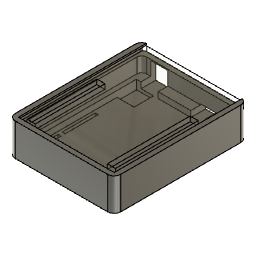
Projet fablabPORCEL (Autodesk Fusion 360 design; units mm, degrees)
Autodesk Fusion 360 part; units mm, degrees
sketch "Esquisse1" plane through (0, 0, 0) normal (0, 0, 1) x (1, 0, 0) in component "boite"
  line L0 (0, 0) -> (65, 0)
  line L1 (65, 0) -> (65, 82)
  line L2 (65, 82) -> (0, 82)
  line L3 (0, 82) -> (0, 0)
  dimension "d4" = 65
  dimension "d5" = 82
  constraint horizontal L0
  constraint vertical L1
  constraint horizontal L2
  constraint vertical L3
  constraint coincident L0.start L3.end
  measures "d4" distance of L0.start L0.end
  measures "d5" distance of L0.start L2.end
extrude "Extrusion1" add sketch "Esquisse1" along normal blind 20 makes body 1 in component "boite"
shell "Coque1" thickness 3 removed faces 1 at (21.6667, 54.6667, 20) on bodies 1 in component "boite"
sketch "Esquisse1 (2)" plane through (0, 0, 3) normal (0, 0, 1) x (-1, 0, 0) in component "boite"
  line L0 (-3, -79) -> (-3, -3)
  line L1 (-3, -3) -> (-62, -3)
  line L2 (-62, -3) -> (-62, -79)
  line L3 (-62, -79) -> (-3, -79)
  line L4 (-59.2367, -6.54) -> (-5.7633, -6.54) construction
  line L5 (-5.7633, -6.54) -> (-5.7633, -72.98)
  line L6 (-5.7633, -72.98) -> (-59.2367, -72.98)
  line L7 (-59.2367, -72.98) -> (-59.2367, -6.54)
  line L8 (-32.5, -6.54) -> (-32.5, -3) construction
  line L9 (-46.1533, -6.54) -> (-43.6133, -4)
  line L10 (-46.1533, -6.54) -> (-53.2911, -6.54) construction
  line L11 (-43.6133, -4) -> (-27.1617, -4)
  line L12 (-27.1617, -4) -> (-27.1617, 3.077) construction
  line L13 (-10.71, -4) -> (-27.1617, -4)
  line L14 (-8.17, -6.54) -> (-10.71, -4)
  line L15 (-59.2367, -6.54) -> (-46.1533, -6.54)
  line L16 (-8.17, -6.54) -> (-5.7633, -6.54)
  line L17 (-57.5967, -7.81) -> (-55.7967, -7.81)
  line L18 (-55.7967, -7.81) -> (-55.7967, -28.13)
  line L19 (-55.7967, -28.13) -> (-57.5967, -28.13)
  line L20 (-57.5967, -28.13) -> (-57.5967, -7.81)
  line L21 (-55.7967, -29.65) -> (-57.5967, -29.65)
  line L22 (-57.5967, -29.65) -> (-57.5967, -55.05)
  line L23 (-57.5967, -55.05) -> (-55.7967, -55.05)
  line L24 (-55.7967, -55.05) -> (-55.7967, -29.65)
  line L25 (-9.2033, -25.59) -> (-7.4033, -25.59)
  line L26 (-7.4033, -25.59) -> (-7.4033, -45.91)
  line L27 (-7.4033, -45.91) -> (-9.2033, -45.91)
  line L28 (-9.2033, -45.91) -> (-9.2033, -25.59)
  line L29 (-37.7367, -5.64) -> (-30.1167, -5.64)
  line L30 (-30.1167, -5.64) -> (-30.1167, -10.72)
  line L31 (-30.1167, -10.72) -> (-37.7367, -10.72)
  line L32 (-37.7367, -10.72) -> (-37.7367, -5.64)
  line L33 (-3.623, -79) -> (-62.17, -79)
  line L34 (-8.5633, -72.98) -> (-19.0633, -72.98)
  line L35 (-19.0633, -72.98) -> (-19.0633, -79)
  line L36 (-19.0633, -79) -> (-8.5633, -79)
  line L37 (-8.5633, -79) -> (-8.5633, -72.98)
  line L38 (-48.2367, -72.98) -> (-39.2367, -72.98)
  line L39 (-39.2367, -72.98) -> (-39.2367, -79)
  line L40 (-39.2367, -79) -> (-48.2367, -79)
  line L41 (-48.2367, -79) -> (-48.2367, -72.98)
  line L42 (-16.2633, -60.98) -> (-5.7633, -60.98)
  line L43 (-5.7633, -60.98) -> (-5.7633, -72.98)
  line L44 (-5.7633, -72.98) -> (-16.2633, -72.98)
  line L45 (-16.2633, -72.98) -> (-16.2633, -60.98)
  line L46 (-7.4033, -7.81) -> (-9.2033, -7.81)
  line L47 (-9.2033, -7.81) -> (-9.2033, -23.05)
  line L48 (-9.2033, -23.05) -> (-7.4033, -23.05)
  line L49 (-7.4033, -23.05) -> (-7.4033, -7.81)
  dimension "d13" = 53.4733
  dimension "d14" = 66.44
  dimension "d20" = 135
  dimension "d21" = 13.0833
  dimension "d22" = 2.54
  dimension "d23" = 16.4517
  dimension "d31" = 2.8
  dimension "d32" = 10.5
  dimension "d33" = 9
  dimension "d34" = 11
  dimension "d43" = 1.27
  dimension "d44" = 1.27
  dimension "d45" = 1.52
  dimension "d46" = 2.54
  dimension "d47" = 1.8
  dimension "d48" = 1.64
  dimension "d49" = 1.64
  dimension "d50" = 20.32
  dimension "d51" = 25.4
  dimension "d52" = 15.24
  dimension "d54" = 12
  dimension "d55" = 10.5
  dimension "d59" = 21.5
  dimension "d60" = 5.08
  dimension "d61" = 7.62
  dimension "d62" = 1.64
  dimension "d102" = 1
  constraint horizontal L4
  constraint vertical L5
  constraint horizontal L6
  constraint vertical L7
  constraint midpoint L4 L8.start
  constraint midpoint L1 L8.end
  constraint parallel L0 L8
  constraint horizontal L10
  constraint coincident L4 L9.start
  constraint horizontal L11
  constraint perpendicular L11 L12
  constraint symmetric L9.start L12 L14.start
  constraint symmetric L9.end L12 L13.start
  constraint symmetric L11.end L12 L13.end
  constraint horizontal L17
  constraint vertical L18
  constraint horizontal L19
  constraint vertical L20
  constraint horizontal L21
  constraint vertical L22
  constraint horizontal L23
  constraint vertical L24
  constraint horizontal L25
  constraint vertical L26
  constraint horizontal L27
  constraint vertical L28
  constraint horizontal L29
  constraint vertical L30
  constraint horizontal L31
  constraint vertical L32
  constraint horizontal L34
  constraint vertical L35
  constraint horizontal L36
  constraint vertical L37
  constraint coincident L33 L35.end
  constraint coincident L6 L34.start
  constraint horizontal L38
  constraint vertical L39
  constraint horizontal L40
  constraint vertical L41
  constraint coincident L33 L39.end
  constraint coincident L6 L38.start
  constraint horizontal L42
  constraint vertical L43
  constraint horizontal L44
  constraint vertical L45
  constraint horizontal L46
  constraint vertical L47
  constraint horizontal L48
  constraint vertical L49
  constraint equal L19 L21
  constraint equal L17 L46
  constraint equal L25 L46
  constraint collinear L18 L24
  constraint collinear L26 L49
  constraint equal L18 L26
  constraint collinear L34 L44
  constraint collinear L5 L43
  constraint parallel L6 L33
  constraint collinear L3 L33
  measures "d13" distance of L4.start L4.end
  measures "d14" distance of L4.start L6.end
  measures "d20" angle of L9 L10
  measures "d21" horizontal distance of L4.start L9.start
  measures "d22" distance of L4 L9.end
  measures "d23" distance of L9.end L11.end
  measures "d31" distance of L5.end L34.start
  measures "d32" distance of L35 L37
  measures "d33" distance of L39 L41
  measures "d34" distance of L7 L41
  measures "d43" distance of L15 L17
  measures "d44" distance of L16 L46
  measures "d45" distance of L19 L21
  measures "d46" distance of L25 L48
  measures "d47" distance of L17.start L17.end
  measures "d48" distance of L7 L20
  measures "d49" distance of L5 L49
  measures "d50" distance of L17 L19
  measures "d51" distance of L21 L23
  measures "d52" distance of L46 L48
  measures "d54" distance of L42.start L44.end
  measures "d55" distance of L42.start L42.end
  measures "d59" distance of L7 L32
  measures "d60" distance of L29.end L30.end
  measures "d61" distance of L29.start L29.end
  measures "d62" distance of L11 L29
  measures "d102" distance of L1 L13
extrude "ExtrusionTrouPin" cut sketch "Esquisse1 (2)" against normal blind 2 contours L5 L6 L34 L42 L43 L44 L45 | L17 L18 L19 L20 | L21 L22 L23 L24 | L25 L26 L27 L28 | L29 L30 L31 L32 | L46 L47 L48 L49 bodies 1 in component "boite"
extrude "ExtrusionSupportArduino" add sketch "Esquisse1 (2)" along normal blind 3.65 contours L0 L1 L2 L3 L5 L6 L7 L9 L11 L13 L14 L15 L16 L33 L37 L41 L43 L44 | L3 L6 L33 L35 L39 bodies 1 in component "boite"
sketch "Esquisse2" plane through (0, 82, 0) normal (0, 1, 0) x (-1, 0, 0) in component "boite"
  line L0 (0, 20) -> (-65, 20)
  line L1 (-65, 0) -> (0, 0)
  line L2 (-63.7, 19) -> (-1.3, 19)
  line L3 (-1.3, 19) -> (-1.3, 15.6)
  line L4 (-1.3, 15.6) -> (-63.7, 15.6)
  line L5 (-63.7, 15.6) -> (-63.7, 19)
  line L6 (-32.5, 19) -> (-32.5, 20) construction
  line L7 (-1.3, 19) -> (-63.7, 19)
  line L8 (-62, 20) -> (-3, 20)
  line L9 (-3, 20) -> (-3, 19)
  line L10 (-3, 19) -> (-62, 19)
  line L11 (-62, 19) -> (-62, 20)
  line L12 (-32.5, 19) -> (-32.5, 20) construction
  line L13 (0, 0) -> (0, 20)
  line L14 (-65, 20) -> (-65, 0)
  dimension "d75" = 3.4
  dimension "d76" = 62.4
  dimension "d79" = 1
  dimension "d119" = 62.4
  dimension "d121" = 59
  constraint horizontal L2
  constraint vertical L3
  constraint horizontal L4
  constraint vertical L5
  constraint midpoint L2 L6.start
  constraint midpoint L0 L6.end
  constraint horizontal L7
  constraint horizontal L8
  constraint vertical L9
  constraint horizontal L10
  constraint vertical L11
  constraint midpoint L10 L6.start
  constraint midpoint L8 L6.end
  constraint perpendicular L8 L12
  constraint collinear L6 L12
  constraint collinear L0 L8
  constraint collinear L2 L10
  measures "d75" distance of L2.end L3.end
  measures "d76" distance of L2.start L2.end
  measures "d79" distance of L0 L2
  measures "d119" distance of L2.end L2.start
  measures "d121" distance of L8.start L8.end
extrude "ExtrusionGlissière" cut sketch "Esquisse2" against normal blind 80.7 contours L2 L3 L4 L5 L7 L10 bodies 1 in component "boite"
extrude "ExtrusionPassageDevantGlissière" cut sketch "Esquisse2" against normal blind 10 contours L0 L2 L7 L8 L9 L10 L11 bodies 1 in component "boite"
fillet "Congé5" radius 4 4 edges at (0, 82, 10) (65, 82, 10) (65, 0, 10) (0, 0, 10) on bodies 1 in component "boite"
fillet "Congé2" radius 3 4 edges at (3, 79, 11.125) (62, 79, 11.125) (62, 3, 11.125) (3, 3, 11.125) on bodies 1 in component "boite"
fillet "Congé4" radius 2 2 edges at (63.7, 1.3, 17.3) (1.3, 1.3, 17.3) on bodies 1 in component "boite"
sketch "Esquisse2 (2)" plane through (0, 79, 0) normal (0, -1, 0) x (1, 0, 0) in component "boite"
  line L0 (59, 6.65) -> (59, 15.6)
  line L1 (59, 15.6) -> (6, 15.6)
  line L2 (6, 15.6) -> (6, 6.65)
  line L3 (6, 6.65) -> (8.5633, 6.65)
  line L4 (19.0633, 3) -> (19.0633, 6.65)
  line L5 (39.2367, 6.65) -> (39.2367, 3)
  line L6 (8.5633, 6.65) -> (8.5633, 3)
  line L7 (19.0633, 6.65) -> (39.2367, 6.65)
  line L8 (39.2367, 3) -> (48.2367, 3)
  line L9 (48.2367, 3) -> (48.2367, 6.65)
  line L10 (48.2367, 6.65) -> (59, 6.65)
  line L11 (59, 6.65) -> (59, 15.6)
  line L12 (59, 15.6) -> (6, 15.6)
  line L13 (6, 15.6) -> (6, 6.65)
  line L14 (6, 6.65) -> (8.5633, 6.65)
  line L15 (8.5633, 6.65) -> (8.5633, 3)
  line L16 (8.5633, 3) -> (19.0633, 3)
  line L17 (19.0633, 3) -> (19.0633, 6.65)
  line L18 (19.0633, 6.65) -> (39.2367, 6.65)
  line L19 (39.2367, 6.65) -> (39.2367, 3)
  line L20 (39.2367, 3) -> (48.2367, 3)
  line L21 (48.2367, 3) -> (48.2367, 6.65)
  line L22 (48.2367, 6.65) -> (59, 6.65)
  line L23 (8.5633, 3) -> (19.0633, 3)
  line L24 (8.5633, 3) -> (19.0633, 3)
  line L25 (19.0633, 3) -> (19.0633, 15)
  line L26 (19.0633, 15) -> (8.5633, 15)
  line L27 (8.5633, 15) -> (8.5633, 3)
  line L28 (48.2367, 3) -> (39.2367, 3)
  line L29 (39.2367, 3) -> (39.2367, 7.2)
  line L30 (39.2367, 7.2) -> (48.2367, 7.2)
  line L31 (48.2367, 7.2) -> (48.2367, 3)
  dimension "d145" = 10.5
  dimension "d146" = 12
  dimension "d147" = 9
  dimension "d148" = 4.2
  constraint horizontal L23
  constraint horizontal L24
  constraint vertical L25
  constraint horizontal L26
  constraint vertical L27
  constraint coincident L6.end L15.end
  constraint horizontal L28
  constraint vertical L29
  constraint horizontal L30
  constraint vertical L31
  measures "d145" distance of L6.end L4.start
  measures "d146" distance of L6.end L26.end
  measures "d147" distance of L8.end L5.end
  measures "d148" distance of L8.end L30.end
extrude "Extrusion5" cut sketch "Esquisse2 (2)" against normal blind 5 contours L5 L8 L9 L19 L20 L21 L28 L29 L30 L31 | L4 L6 L15 L16 L17 L23 L24 L25 L26 L27 bodies 1 in component "boite"
sketch "Esquisse1 (3)" plane through (0, 0, 3) normal (0, 0, 1) x (-1, 0, 0) in component "vitre"
  line L0 (25, -1) -> (87, -1)
  line L1 (87, -1) -> (87, -81.5)
  line L2 (87, -81.5) -> (25, -81.5)
  line L3 (25, -81.5) -> (25, -1)
  line L4 (-48.2367, -72.98) -> (-48.2367, -82)
  line L5 (-48.2367, -82) -> (-39.2367, -82)
  line L6 (-39.2367, -82) -> (-39.2367, -72.98)
  line L7 (-39.2367, -72.98) -> (-19.0633, -72.98)
  line L8 (-19.0633, -72.98) -> (-19.0633, -82)
  line L9 (-19.0633, -82) -> (-8.5633, -82)
  line L10 (-8.5633, -82) -> (-8.5633, -72.98)
  line L11 (-8.5633, -72.98) -> (-16.2633, -72.98)
  line L12 (-16.2633, -72.98) -> (-16.2633, -60.98)
  line L13 (-16.2633, -60.98) -> (-5.7633, -60.98)
  line L14 (-5.7633, -60.98) -> (-5.7633, -6.54)
  line L15 (-5.7633, -6.54) -> (-8.17, -6.54)
  line L16 (-8.17, -6.54) -> (-10.71, -4)
  line L17 (-10.71, -4) -> (-43.6133, -4)
  line L18 (-43.6133, -4) -> (-46.1533, -6.54)
  line L19 (-46.1533, -6.54) -> (-59.2367, -6.54)
  line L20 (-59.2367, -6.54) -> (-59.2367, -72.98)
  line L21 (-59.2367, -72.98) -> (-48.2367, -72.98)
  line L22 (-57.5967, -29.65) -> (-55.7967, -29.65)
  line L23 (-55.7967, -29.65) -> (-55.7967, -55.05)
  line L24 (-55.7967, -55.05) -> (-57.5967, -55.05)
  line L25 (-57.5967, -55.05) -> (-57.5967, -29.65)
  line L26 (-30.1167, -5.64) -> (-30.1167, -10.72)
  line L27 (-30.1167, -10.72) -> (-37.7367, -10.72)
  line L28 (-37.7367, -10.72) -> (-37.7367, -5.64)
  line L29 (-37.7367, -5.64) -> (-30.1167, -5.64)
  line L30 (-9.2033, -7.81) -> (-7.4033, -7.81)
  line L31 (-7.4033, -7.81) -> (-7.4033, -23.05)
  line L32 (-7.4033, -23.05) -> (-9.2033, -23.05)
  line L33 (-9.2033, -23.05) -> (-9.2033, -7.81)
  line L34 (-55.7967, -7.81) -> (-55.7967, -28.13)
  line L35 (-55.7967, -28.13) -> (-57.5967, -28.13)
  line L36 (-57.5967, -28.13) -> (-57.5967, -7.81)
  line L37 (-57.5967, -7.81) -> (-55.7967, -7.81)
  line L38 (-7.4033, -25.59) -> (-7.4033, -45.91)
  line L39 (-7.4033, -45.91) -> (-9.2033, -45.91)
  line L40 (-9.2033, -45.91) -> (-9.2033, -25.59)
  line L41 (-9.2033, -25.59) -> (-7.4033, -25.59)
  dimension "d85" = 62
  dimension "d86" = 80.5
  dimension "d99" = 25
  dimension "d100" = 1
  constraint horizontal L0
  constraint vertical L1
  constraint horizontal L2
  constraint vertical L3
  measures "d85" distance of L0.start L0.end
  measures "d86" distance of L0.start L2.end
  measures "d99" distance of origin L3
  measures "d100" distance of origin L0
extrude "Extrusion1'" add sketch "Esquisse1 (3)" along normal blind 3 separate body contours L0 L1 L2 L3 makes body 2 in component "vitre"
fillet "Congé2'" radius 2 4 edges at (-25, 81.5, 4.5) (-87, 81.5, 4.5) (-87, 1, 4.5) (-25, 1, 4.5) on bodies 2 in component "vitre"
sketch "Esquisse5" plane through (-88.5, 0, -10) normal (0, 0, 1) x (-1, 0, 0) in component "vitre"
  line L0 (-5.7633, -5.54) -> (-10.7633, -5.54)
  line L1 (-10.7633, -5.54) -> (-10.7633, -48.54)
  line L2 (-10.7633, -48.54) -> (-5.7633, -48.54)
  line L3 (-5.7633, -48.54) -> (-5.7633, -5.54)
  line L4 (-16.2633, -72.98) -> (-16.2633, -60.98)
  line L5 (-16.2633, -60.98) -> (-5.7633, -60.98)
  line L6 (-57.5967, -29.65) -> (-55.7967, -29.65)
  line L7 (-55.7967, -29.65) -> (-55.7967, -55.05)
  line L8 (-55.7967, -55.05) -> (-57.5967, -55.05)
  line L9 (-57.5967, -55.05) -> (-57.5967, -29.65)
  line L10 (-30.1167, -5.64) -> (-30.1167, -10.72)
  line L11 (-30.1167, -10.72) -> (-37.7367, -10.72)
  line L12 (-37.7367, -10.72) -> (-37.7367, -5.64)
  line L13 (-37.7367, -5.64) -> (-30.1167, -5.64)
  line L14 (-9.2033, -7.81) -> (-7.4033, -7.81)
  line L15 (-7.4033, -7.81) -> (-7.4033, -23.05)
  line L16 (-7.4033, -23.05) -> (-9.2033, -23.05)
  line L17 (-9.2033, -23.05) -> (-9.2033, -7.81)
  line L18 (-55.7967, -7.81) -> (-55.7967, -28.13)
  line L19 (-55.7967, -28.13) -> (-57.5967, -28.13)
  line L20 (-57.5967, -28.13) -> (-57.5967, -7.81)
  line L21 (-57.5967, -7.81) -> (-55.7967, -7.81)
  line L22 (-7.4033, -25.59) -> (-7.4033, -45.91)
  line L23 (-7.4033, -45.91) -> (-9.2033, -45.91)
  line L24 (-9.2033, -45.91) -> (-9.2033, -25.59)
  line L25 (-9.2033, -25.59) -> (-7.4033, -25.59)
  line L26 (-48.2367, -72.98) -> (-48.2367, -82)
  line L27 (-48.2367, -82) -> (-39.2367, -82)
  line L28 (-39.2367, -82) -> (-39.2367, -72.98)
  line L29 (-39.2367, -72.98) -> (-19.0633, -72.98)
  line L30 (-19.0633, -72.98) -> (-19.0633, -82)
  line L31 (-19.0633, -82) -> (-8.5633, -82)
  line L32 (-8.5633, -82) -> (-8.5633, -72.98)
  line L33 (-8.5633, -72.98) -> (-16.2633, -72.98)
  line L34 (-5.7633, -60.98) -> (-5.7633, -6.54)
  line L35 (-5.7633, -6.54) -> (-8.17, -6.54)
  line L36 (-8.17, -6.54) -> (-10.71, -4)
  line L37 (-10.71, -4) -> (-43.6133, -4)
  line L38 (-43.6133, -4) -> (-46.1533, -6.54)
  line L39 (-46.1533, -6.54) -> (-59.2367, -6.54)
  line L40 (-59.2367, -6.54) -> (-59.2367, -72.98)
  line L41 (-59.2367, -72.98) -> (-48.2367, -72.98)
  line L42 (-59.2367, -6.54) -> (-5.7633, -6.54)
  line L43 (-5.7633, -6.54) -> (-5.7633, -72.98)
  line L44 (-48.2367, -72.98) -> (-48.2367, -82)
  line L45 (-48.2367, -82) -> (-39.2367, -82)
  line L46 (-39.2367, -82) -> (-39.2367, -72.98)
  line L47 (-39.2367, -72.98) -> (-19.0633, -72.98)
  line L48 (-19.0633, -72.98) -> (-19.0633, -82)
  line L49 (-19.0633, -82) -> (-8.5633, -82)
  line L50 (-8.5633, -82) -> (-8.5633, -72.98)
  line L51 (-8.5633, -72.98) -> (-16.2633, -72.98)
  line L52 (-16.2633, -72.98) -> (-16.2633, -60.98)
  line L53 (-16.2633, -60.98) -> (-5.7633, -60.98)
  line L54 (-5.7633, -60.98) -> (-5.7633, -6.54)
  line L55 (-5.7633, -6.54) -> (-8.17, -6.54)
  line L56 (-8.17, -6.54) -> (-10.71, -4)
  line L57 (-10.71, -4) -> (-43.6133, -4)
  line L58 (-43.6133, -4) -> (-46.1533, -6.54)
  line L59 (-46.1533, -6.54) -> (-59.2367, -6.54)
  line L60 (-59.2367, -6.54) -> (-59.2367, -72.98)
  line L61 (-59.2367, -72.98) -> (-48.2367, -72.98)
  line L62 (-57.5967, -29.65) -> (-55.7967, -29.65)
  line L63 (-55.7967, -29.65) -> (-55.7967, -55.05)
  line L64 (-55.7967, -55.05) -> (-57.5967, -55.05)
  line L65 (-57.5967, -55.05) -> (-57.5967, -29.65)
  line L66 (-30.1167, -5.64) -> (-30.1167, -10.72)
  line L67 (-30.1167, -10.72) -> (-37.7367, -10.72)
  line L68 (-37.7367, -10.72) -> (-37.7367, -5.64)
  line L69 (-37.7367, -5.64) -> (-30.1167, -5.64)
  line L70 (-9.2033, -7.81) -> (-7.4033, -7.81)
  line L71 (-7.4033, -7.81) -> (-7.4033, -23.05)
  line L72 (-7.4033, -23.05) -> (-9.2033, -23.05)
  line L73 (-9.2033, -23.05) -> (-9.2033, -7.81)
  line L74 (-55.7967, -7.81) -> (-55.7967, -28.13)
  line L75 (-55.7967, -28.13) -> (-57.5967, -28.13)
  line L76 (-57.5967, -28.13) -> (-57.5967, -7.81)
  line L77 (-57.5967, -7.81) -> (-55.7967, -7.81)
  line L78 (-7.4033, -25.59) -> (-7.4033, -45.91)
  line L79 (-7.4033, -45.91) -> (-9.2033, -45.91)
  line L80 (-9.2033, -45.91) -> (-9.2033, -25.59)
  line L81 (-9.2033, -25.59) -> (-7.4033, -25.59)
  line L82 (-48.2367, -72.98) -> (-48.2367, -82)
  line L83 (-48.2367, -82) -> (-39.2367, -82)
  line L84 (-39.2367, -82) -> (-39.2367, -72.98)
  line L85 (-39.2367, -72.98) -> (-19.0633, -72.98)
  line L86 (-19.0633, -72.98) -> (-19.0633, -82)
  line L87 (-19.0633, -82) -> (-8.5633, -82)
  line L88 (-8.5633, -82) -> (-8.5633, -72.98)
  line L89 (-8.5633, -72.98) -> (-16.2633, -72.98)
  line L90 (-16.2633, -72.98) -> (-16.2633, -60.98)
  line L91 (-16.2633, -60.98) -> (-5.7633, -60.98)
  line L92 (-5.7633, -60.98) -> (-5.7633, -6.54)
  line L93 (-5.7633, -6.54) -> (-8.17, -6.54)
  line L94 (-8.17, -6.54) -> (-10.71, -4)
  line L95 (-10.71, -4) -> (-43.6133, -4)
  line L96 (-43.6133, -4) -> (-46.1533, -6.54)
  line L97 (-46.1533, -6.54) -> (-59.2367, -6.54)
  line L98 (-59.2367, -6.54) -> (-59.2367, -72.98)
  line L99 (-59.2367, -72.98) -> (-48.2367, -72.98)
  line L100 (-57.5967, -29.65) -> (-55.7967, -29.65)
  line L101 (-55.7967, -29.65) -> (-55.7967, -55.05)
  line L102 (-55.7967, -55.05) -> (-57.5967, -55.05)
  line L103 (-57.5967, -55.05) -> (-57.5967, -29.65)
  line L104 (-30.1167, -5.64) -> (-30.1167, -10.72)
  line L105 (-30.1167, -10.72) -> (-37.7367, -10.72)
  line L106 (-37.7367, -10.72) -> (-37.7367, -5.64)
  line L107 (-37.7367, -5.64) -> (-30.1167, -5.64)
  line L108 (-9.2033, -7.81) -> (-7.4033, -7.81)
  line L109 (-7.4033, -7.81) -> (-7.4033, -23.05)
  line L110 (-7.4033, -23.05) -> (-9.2033, -23.05)
  line L111 (-9.2033, -23.05) -> (-9.2033, -7.81)
  line L112 (-55.7967, -7.81) -> (-55.7967, -28.13)
  line L113 (-55.7967, -28.13) -> (-57.5967, -28.13)
  line L114 (-57.5967, -28.13) -> (-57.5967, -7.81)
  line L115 (-57.5967, -7.81) -> (-55.7967, -7.81)
  line L116 (-7.4033, -25.59) -> (-7.4033, -45.91)
  line L117 (-7.4033, -45.91) -> (-9.2033, -45.91)
  line L118 (-9.2033, -45.91) -> (-9.2033, -25.59)
  line L119 (-9.2033, -25.59) -> (-7.4033, -25.59)
  line L120 (-54.2367, -57.54) -> (-59.2367, -57.54)
  line L121 (-59.2367, -57.54) -> (-59.2367, -5.54)
  line L122 (-59.2367, -5.54) -> (-54.2367, -5.54)
  line L123 (-54.2367, -5.54) -> (-54.2367, -57.54)
  line L124 (-59.2367, -72.98) -> (-59.2367, -6.54)
  dimension "d132" = 5
  dimension "d133" = 43
  dimension "d153" = 1
  dimension "d154" = 5
  dimension "d155" = 52
  constraint horizontal L0
  constraint vertical L1
  constraint horizontal L2
  constraint vertical L3
  constraint collinear L3 L43
  constraint horizontal L120
  constraint vertical L121
  constraint horizontal L122
  constraint vertical L123
  constraint collinear L121 L124
  constraint collinear L0 L122
  measures "d132" distance of L0.start L0.end
  measures "d133" distance of L0.start L2.end
  measures "d153" distance of L0 L42
  measures "d154" distance of L121.end L122.end
  measures "d155" distance of L120.start L122.end
extrude "Extrusion2" cut sketch "Esquisse5" along normal blind 22 contours L0 L3 L35 L36 L42 L55 L56 L93 L94 | L0 L1 L36 L42 L56 L94 | L1 L2 L3 L34 L35 L42 L43 L54 L55 L92 L93 | L39 L40 L42 L59 L60 L97 L98 L120 L121 L123 L124 | L6 L7 L8 L9 L62 L63 L64 L65 L100 L101 L102 L103 | L14 L15 L16 L17 L70 L71 L72 L73 L108 L109 L110 L111 | L18 L19 L20 L21 L74 L75 L76 L77 L112 L113 L114 L115 | L22 L23 L24 L25 L78 L79 L80 L81 L116 L117 L118 L119 bodies 2 in component "vitre"
component "boite" placed x (1, 0, 0) y (0, 1, 0) z (0, 0, 1) at (0, 0, 0)
component "vitre" placed x (1, 0, 0) y (0, 1, 0) z (0, 0, 1) at (88.5, 0, 13)
equation "longueurBoite = 82 mm"
equation "largeurBoite = 65 mm"
equation "hauteurBoite = 20 mm"
equation "d4 = largeurBoite"
equation "d5 = longueurBoite"
equation "longueurArduino = 66.04 mm + marge"
equation "d7 = hauteurBoite"
equation "d9 = epaisseur"
equation "largeurArduino = 53.34 mm + ( marge / 3 mm ) * 1 mm"
equation "d13 = largeurArduino"
equation "d14 = longueurArduino"
equation "largeurArduino2 = 12.95 mm + marge / 3" comment "l'arduino n'est pas un rectangle, c'est pour faire sa déformation"
equation "angleArduino = 135 deg" comment "l'arduino n'est pas un rectangle, c'est pour faire sa déformation"
equation "largeurArduino3 = 32.77 mm + ( marge / 3 mm ) * 1 mm" comment "l'arduino n'est pas un rectangle, c'est pour faire sa déformation"
equation "longueurArduino2 = 2.54 mm" comment "l'arduino n'est pas un rectangle, c'est pour faire sa déformation"
equation "d20 = angleArduino"
equation "d21 = largeurArduino2"
equation "d22 = longueurArduino2"
equation "d23 = largeurArduino3 / 2"
equation "distanceAlim = 2.8 mm"
equation "largAlim = 10.5 mm"
equation "distanceUSB = 11 mm"
equation "largUSB = 9 mm"
equation "epaisseur = 3 mm" comment "pour le support de la carte et pour la boîte"
equation "d31 = distanceAlim"
equation "d32 = largAlim"
equation "d33 = largUSB"
equation "d34 = distanceUSB"
equation "longPin1GET2D = 20.32 mm" comment "longueur du 1er pin de gauche et du deuxième pin de droite"
equation "distancePin1 = 1.27 mm" comment "distance entre le pin 1 gauche et droite et et le bord du support de la carte"
equation "distancePin2G = 1.52 mm"
equation "distancePin2D = 2.54 mm"
equation "longPin2G = 25.4 mm"
equation "lonPin1D = 15.24 mm"
equation "largeurPin = 1.8 mm"
equation "distLargPin = 2.54 mm - largeurPin / 2"
equation "d43 = distancePin1"
equation "d44 = distancePin1"
equation "d45 = distancePin2G"
equation "d46 = distancePin2D"
equation "d47 = largeurPin"
equation "d48 = distLargPin"
equation "d49 = distLargPin"
equation "d50 = longPin1GET2D"
equation "d51 = longPin2G"
equation "d52 = lonPin1D"
equation "hautPinAlim = 12 mm"
equation "d55 = largAlim"
equation "distancePinM = 21.5 mm" comment "la distance des pins du milieu"
equation "larPinM = 7.62 mm"
equation "longPinM = 5.08 mm"
equation "d59 = distancePinM"
equation "d60 = longPinM"
equation "d61 = larPinM"
equation "d62 = distLargPin"
equation "hauteurSupportCarte = 1.65 mm + 2 mm" comment "hauteur de la carte : 1.65"
equation "profondeurPin = 2 mm"
equation "d70 = congéInter"
equation "longVitre = longueurBoite - epaisseur"
equation "largVitre = largeurBoite - epaisseur"
equation "hauteurVitre = 3 mm"
equation "distanceVitre = 1 mm" comment "distance entre le haut de la vitre et le haut de la boite"
equation "d75 = hauteurVitre + marge"
equation "d76 = largVitre + marge"
equation "d79 = distanceVitre"
equation "d81 = -longueurBoite + ( largeurBoite - largVitre - marge ) / 2"
equation "d85 = largVitre"
equation "d86 = longVitre + ( largeurBoite - largVitre ) / 2"
equation "d87 = hauteurVitre"
equation "marge = 0.4 mm"
equation "d102 = positionArduinoDansLaBoite"
equation "positionArduinoDansLaBoite = 1 mm"
equation "hauteurAlim = 12 mm"
equation "hauteurUSB = 4.2 mm"
equation "d119 = largVitre + marge"
equation "d121 = largeurBoite - 2 * epaisseur"
equation "congéVitre = 2 mm"
equation "d128 = congéVitre"
equation "trouDroiteVitreLong = 43 mm"
equation "trouGaucheVitreLong = 52 mm"
equation "trouVitreLarg = 5 mm"
equation "d132 = trouVitreLarg"
equation "d133 = trouDroiteVitreLong"
equation "d141 = -profondeurPin"
equation "d143 = hauteurSupportCarte"
equation "d145 = largAlim"
equation "d146 = hauteurAlim"
equation "d147 = largUSB"
equation "d148 = hauteurUSB"
equation "d150 = congéVitre"
equation "d152 = congéContour"
equation "d154 = trouVitreLarg"
equation "d155 = trouGaucheVitreLong"
equation "congéContour = 4 mm"
equation "congéInter = 3 mm"
